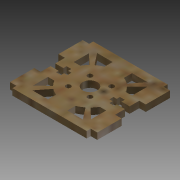
# Autodesk Inventor part: MotorSupport
Saved by Autodesk Inventor 2012 (Build 160160000, 160)
## iProperties
Created: 2014-07-10
Part Number: MotorSupport
Material: Default
Document SubType Name: Modeling
Designer: Anon
Density: 1 g/cm^3
Author: Anon
Autodesk Inventor part; units mm, degrees
ref_plane "YZ Plane" through (0, 0, 0) normal (1, 0, 0) x (0, 1, 0)
ref_plane "XZ Plane" through (0, 0, 0) normal (0, 1, 0) x (-1, 0, 0)
ref_plane "XY Plane" through (0, 0, 0) normal (0, 0, 1) x (1, 0, 0)
sketch "Sketch1" plane through (0, 0, 0) normal (0, 0, 1) x (1, 0, 0)
  line L0 (-27, 25) -> (27, 25)
  line L1 (27, 25) -> (27, -25)
  line L2 (27, -25) -> (-27, -25)
  line L3 (-27, -25) -> (-27, 25)
  point P0 (0, 0)
  dimension "d0" = 54
  dimension "d1" = 50
  dimension "d2" = 25
  dimension "d3" = 27
  constraints: 8 end point, 2 parallel, 1 horizontal, 1 perpendicular
  measures "d0" distance of L1.end L2.end
  measures "d1" distance of L0.end L1.end
  measures "d2" distance from line of L0 point (0, 0)
  measures "d3" distance from line of L3 point (0, 0)
extrude "Base" add sketch "Sketch1" along normal blind 4
sketch "Sketch2" plane through (0, 0, 4) normal (0, 0, 1) x (1, 0, 0)
  line L0 (-27, -25) -> (-27, 25) projected
  line L1 (0, 23.0221) -> (0, -15.4934) construction
  line L2 (-23.6958, 0) -> (15.7708, 0) construction
  line L3 (-27, 7.5) -> (-23, 7.5)
  line L4 (-23, 7.5) -> (-23, -7.5)
  line L5 (-23, -7.5) -> (-27, -7.5)
  line L6 (-27, -7.5) -> (-27, 7.5)
  line L7 (-27, 25) -> (-23, 25)
  line L8 (-23, 25) -> (-23, 22.5)
  line L9 (-23, 22.5) -> (-27, 22.5)
  line L10 (-27, 22.5) -> (-27, 25)
  line L11 (-27, -25) -> (-23, -25)
  line L12 (-23, -25) -> (-23, -22.5)
  line L13 (-23, -22.5) -> (-27, -22.5)
  line L14 (-27, -22.5) -> (-27, -25)
  line L15 (27, 7.5) -> (23, 7.5)
  line L16 (23, 7.5) -> (23, -7.5)
  line L17 (23, -7.5) -> (27, -7.5)
  line L18 (27, -7.5) -> (27, 7.5)
  line L19 (27, 25) -> (23, 25)
  line L20 (23, 25) -> (23, 22.5)
  line L21 (23, 22.5) -> (27, 22.5)
  line L22 (27, 22.5) -> (27, 25)
  line L23 (27, -25) -> (23, -25)
  line L24 (23, -25) -> (23, -22.5)
  line L25 (23, -22.5) -> (27, -22.5)
  line L26 (27, -22.5) -> (27, -25)
  point P0 (0, 0)
  point P1 (23.6958, 0)
  dimension "d9" = 4
  dimension "d10" = 15
  dimension "d11" = 4
  dimension "d13" = 7.5
  dimension "d14" = 15
  dimension "d15" = 15
  dimension "d16" = 4
  constraints: 52 end point, 11 symmetric about line, 6 parallel, 4 perpendicular, 3 horizontal, 1 point on line
  measures "d9" distance of L4.end L5.end
  measures "d10" distance of L3.end L4.end
  measures "d11" distance of L8.end L9.end
  measures "d13" distance from line of point (0, 0) L3
  measures "d14" distance between parallel lines of L3 L9
  measures "d15" distance between parallel lines of L13 L5
  measures "d16" distance between parallel lines of L0 L12
extrude "Sleeves" cut sketch "Sketch2" against normal blind 4
sketch "Sketch3" plane through (0, 0, 4) normal (0, 0, 1) x (1, 0, 0)
  line L0 (0, 0) -> (-5.6569, 5.6569) construction
  line L1 (0, 0) -> (8, 0) construction
  line L2 (0, 0) -> (6.7175, 6.7175) construction
  line L3 (0, 0) -> (-6.7175, -6.7175) construction
  line L4 (0, 0) -> (5.6569, -5.6569) construction
  dimension "d19" = 8
  dimension "d20" = 135
  dimension "d21" = 9.5
  dimension "d22" = 9.5
  dimension "d23" = 8
  constraints: 10 end point, 4 coincident, 2 perpendicular, 1 collinear, 1 equal length, 1 horizontal
  measures "d19" distance of L0.start L0.end
  measures "d20" angle of L1 L0
  measures "d21" distance of L0.start L2.end
  measures "d22" distance of L0.start L3.end
  measures "d23" distance of L0.start L4.end
hole "MotorMounts" at (6.7175, 6.7175, 4) at (-5.6569, 5.6569, 4) at (-6.7175, -6.7175, 4) at (5.6569, -5.6569, 4) direction (0, 0, -1) diameter 3 end through all
sketch "Sketch4" plane through (0, 0, 4) normal (0, 0, 1) x (1, 0, 0)
  circle A0 centre (0, 0) radius 4.5
  dimension "d31" = 9
  constraints: 1 centre point, 1 coincident
  measures "d31" diameter of A0
extrude "ShaftClearance" cut sketch "Sketch4" against normal through all
sketch "Sketch5" plane through (0, 0, 4) normal (0, 0, 1) x (1, 0, 0)
  circle A0 centre (0, 0) radius 4.5 projected
  line L0 (-23, 7.5) -> (-23, -7.5) projected
  line L1 (23, -7.5) -> (23, 7.5) projected
  line L2 (-23, 1.5) -> (-18, 1.5)
  line L3 (-18, 1.5) -> (-18, 3.5)
  line L4 (-18, 3.5) -> (-15, 3.5)
  line L5 (-15, 3.5) -> (-15, 1.5)
  line L6 (-15, 1.5) -> (-13, 1.5)
  line L7 (-13, 1.5) -> (-13, -1)
  line L8 (-13, -1) -> (-15, -1)
  line L9 (-15, -1) -> (-15, -3)
  line L10 (-15, -3) -> (-18, -3)
  line L11 (-18, -3) -> (-18, -1.4035)
  line L12 (-18, -1.4035) -> (-23, -1.4035)
  line L13 (-23, -1.4035) -> (-23, 1.5)
  dimension "d34" = 5
  dimension "d35" = 2
  dimension "d36" = 3
  dimension "d37" = 2
  dimension "d38" = 2.5
  dimension "d39" = 2
  dimension "d40" = 3
  dimension "d41" = 1.5
  constraints: 24 end point, 5 parallel, 5 perpendicular, 2 collinear, 2 point on line
  measures "d34" distance of L2.start L2.end
  measures "d35" distance of L2.end L3.end
  measures "d36" distance of L3.end L4.end
  measures "d37" distance of L5.end L6.end
  measures "d38" distance of L6.end L7.end
  measures "d39" distance of L8.end L9.end
  measures "d40" distance of L9.end L10.end
  measures "d41" distance from line of A0.centre L2
extrude "ScrewLock" cut sketch "Sketch5" against normal blind 10 contours L2 L3 L4 L5 L6 L7 L8 L9 L10 L11 L12 L0
mirror "ScrewLockDoubler" about plane through (0, 0, 0) normal (1, 0, 0) of "ScrewLock"
sketch "Sketch6" plane through (0, 0, 4) normal (0, 0, 1) x (1, 0, 0)
  line L0 (-23, 25) -> (23, 25) projected
  line L1 (-23, 25) -> (-23, 22.5) projected
  line L2 (18, 3.5) -> (18, 1.5) projected
  line L3 (-18, 20) -> (-6, 20)
  line L4 (-6, 20) -> (-6, 15)
  line L5 (-18, 20) -> (-18, 8)
  line L6 (15, 3.5) -> (18, 3.5) projected
  circle A0 centre (0, 0) radius 4.5 projected
  arc A1 (-6, 15) -> (-14.0357, 8) centre (0, 0) ccw
  line L7 (-14.0357, 8) -> (-18, 8)
  dimension "d44" = 5
  dimension "d45" = 12
  dimension "d46" = 12
  dimension "d48" = 5
  dimension "d49" = 5
  constraints: 8 end point, 2 parallel, 2 perpendicular, 2 point on circle, 1 centre point, 1 coincident
  measures "d44" distance of L3.end L4.end
  measures "d45" distance of L3.start L3.end
  measures "d46" distance of L3.start L5.end
  measures "d48" distance between parallel lines of L0 L3
  measures "d49" distance between parallel lines of L1 L5
extrude "CornerCutout" cut sketch "Sketch6" against normal blind 10 contours L3 L4 A1 L7 L5
sketch "Sketch7" plane through (0, 0, 4) normal (0, 0, 1) x (1, 0, 0)
  line L0 (-18, 8) -> (-18, 20) projected
  line L1 (-18, 20) -> (-6, 20) projected
  arc A0 (-6, 15) -> (-14.0357, 8) centre (0, 0) ccw projected
  line L2 (18, 3.5) -> (18, 1.5) projected
  circle A1 centre (0, 0) radius 4.5 projected
  line L3 (0, 0) -> (-18.1317, 23.2182) construction
  line L4 (0, 0) -> (-21.2105, 20.4919) construction
  line L5 (0, 0) -> (-18, 20) construction
  line L6 (-15.6185, 20) -> (-9.9435, 12.7329)
  line L7 (-15.6185, 20) -> (-18, 20)
  line L8 (-18, 17.3902) -> (-18, 20)
  line L9 (-18, 17.3902) -> (-11.6188, 11.2251)
  arc A2 (-9.9435, 12.7329) -> (-11.6188, 11.2251) centre (0, 0) ccw
  dimension "d52" = 8
  dimension "d54" = 4
  constraints: 14 end point, 6 point on line, 4 point on circle, 2 perpendicular, 1 centre point, 1 coincident
  measures "d52" angle of L3 L4
  measures "d54" angle of L3 L5
extrude "DiagonalSupport" add sketch "Sketch7" against normal blind 4 contours L0 L1 L6 A0 L9
mirror "CornerDoubler" about plane through (0, 0, 0) normal (0, 1, 0) of "CornerCutout", "DiagonalSupport"
mirror "CornerQuadrupler" about plane through (0, 0, 0) normal (1, 0, 0) of "CornerCutout", "CornerDoubler", "DiagonalSupport"
body "Solid1"
